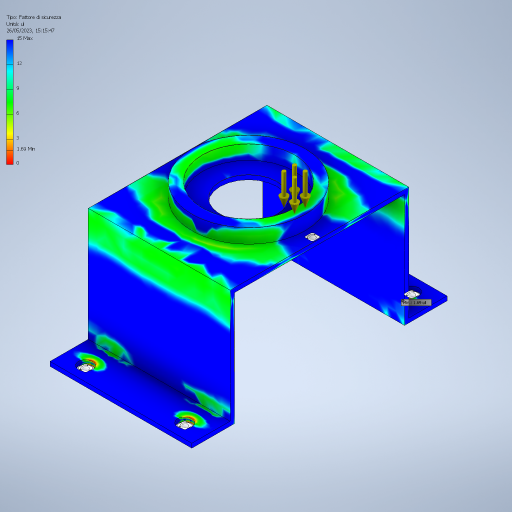
# Autodesk Inventor part: Sanson_Amedeo Analisi FEM 2
Saved by Autodesk Inventor 2023 (Build 270158000, 158)
## iProperties
Created: 2023-05-26
Part Number: Sanson_Amedeo Analisi FEM 2
Material: Generico
Document SubType Name: Modeling
Designer: Admin
Mass: 136.395 g
Surface Area: 717.234 cm^2
Volume: 136.395 cm^3
Density: 1 g/cm^3
Appearance: Default
Author: Admin
Autodesk Inventor part; units mm, degrees
ref_plane "YZ Plane" through (0, 0, 0) normal (1, 0, 0) x (0, 1, 0)
ref_plane "XZ Plane" through (0, 0, 0) normal (0, 1, 0) x (-1, 0, 0)
ref_plane "XY Plane" through (0, 0, 0) normal (0, 0, 1) x (1, 0, 0)
sketch "Schizzo1" plane through (0, 0, 0) normal (1, 0, 0) x (0, 1, 0)
  line L0 (0, 90) -> (0, 60)
  line L1 (0, 60) -> (80, 60)
  line L2 (80, 60) -> (80, -60)
  line L3 (80, -60) -> (0, -60)
  line L4 (0, -60) -> (0, -90)
  line L5 (0, -90) -> (3, -90)
  line L6 (3, -90) -> (3, -63)
  line L7 (3, -63) -> (83, -63)
  line L8 (83, -63) -> (83, 63)
  line L9 (83, 63) -> (3, 63)
  line L10 (3, 63) -> (3, 90)
  line L11 (3, 90) -> (0, 90)
  line L12 (0, 0) -> (59.7399, 0) construction
  line L13 (0, 0) -> (0, -69.3642) construction
  dimension "d0" = 30
  dimension "d1" = 120
  dimension "d2" = 3
  dimension "d3" = 3
  dimension "d4" = 83
  dimension "d5" = 3
  constraints: 28 end point, 9 perpendicular, 4 point on line, 2 vertical, 1 horizontal, 4 other
  measures "d0" distance of L0.start L0.end
  measures "d1" distance of L1.end L2.end
  measures "d2" distance between parallel lines of L7 L3
  measures "d3" distance between parallel lines of L2 L8
  measures "d4" distance between parallel lines of L8 L4
  measures "d5" distance between parallel lines of L4 L6
extrude "Estrusione1" add sketch "Schizzo1" along normal mid plane 100
sketch "Schizzo2" plane through (-50, 83, 63) normal (0, 1, 0) x (1, 0, 0)
  circle A0 centre (50, 63) radius 40
  circle A1 centre (50, 63) radius 32.5
  circle A2 centre (50, 63) radius 20
  dimension "d8" = 80
  dimension "d9" = 65
  dimension "d10" = 40
  constraints: 3 centre point, 3 coincident
  measures "d8" diameter of A0
  measures "d9" diameter of A1
  measures "d10" diameter of A2
extrude "Estrusione2" cut sketch "Schizzo2" against normal through all contours A2
extrude "Estrusione3" add sketch "Schizzo2" along normal blind 10 contours A0
sketch "Schizzo3" plane through (-50, 3, 90) normal (0, 1, 0) x (1, 0, 0)
  line L0 (100, 0) -> (100, 30) projected
  line L1 (100, 30) -> (0, 30) projected
  line L2 (0, 150) -> (100, 150) projected
  line L3 (100, 150) -> (100, 180) projected
  line L4 (0, 180) -> (100, 180) projected
  line L5 (0, 0) -> (100, 0) projected
  line L6 (0, 30) -> (0, 0) projected
  line L7 (0, 180) -> (0, 150) projected
  line L8 (100, 0) -> (85, 0)
  line L9 (85, 0) -> (85, 10)
  circle A0 centre (85, 10) radius 5
  circle A1 centre (85, 170) radius 5
  circle A2 centre (15, 10) radius 5
  circle A3 centre (15, 170) radius 5
  point P0 (50, 90)
  dimension "d15" = 15
  dimension "d16" = 10
  dimension "d17" = 10
  dimension "d20" = 160
  dimension "d23" = 70
  constraints: 4 centre point, 4 end point, 1 coincident, 1 horizontal, 1 perpendicular, 1 point on line, 1 vertical, 6 other
  measures "d15" distance of L0.start L8.end
  measures "d16" distance of L8.end L9.end
  measures "d17" diameter of A0
  measures "d20" distance of A0.centre A1.centre
  measures "d23" distance of A0.centre A2.centre
extrude "Estrusione4" cut sketch "Schizzo3" against normal through all contours A0 | A1 | A2 | A3
sketch "Schizzo4" plane through (-50, 3, 90) normal (0, 1, 0) x (1, 0, 0)
  point P0 (50, 90)
sketch "Schizzo5" plane through (-50, 3, 90) normal (0, 1, 0) x (1, 0, 0)
  point P0 (50, 90)
